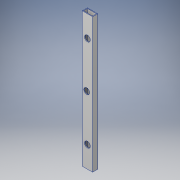
# Autodesk Inventor part: 26in 2x1
Saved by Autodesk Inventor 2018 (Build 220112000, 112)
## iProperties
Created: 2018-01-13
Part Number: 26in 2x1
Material: Aluminum 6061
Document SubType Name: Modeling
Designer: maste
Density: 2.7 g/cm^3
Appearance: Aluminum - Flat
Author: maste
Autodesk Inventor part; units mm, degrees
ref_plane "YZ Plane" through (0, 0, 0) normal (1, 0, 0) x (0, 1, 0)
ref_plane "XZ Plane" through (0, 0, 0) normal (0, 1, 0) x (-1, 0, 0)
ref_plane "XY Plane" through (0, 0, 0) normal (0, 0, 1) x (1, 0, 0)
sketch "Sketch1" plane through (0, 0, 0) normal (0, 1, 0) x (-1, 0, 0)
  line L0 (0, 0) -> (-50.8, 0)
  line L1 (-50.8, 0) -> (-50.8, -25.4)
  line L2 (-50.8, -25.4) -> (0, -25.4)
  line L3 (0, -25.4) -> (0, 0)
  line L4 (-3.175, -22.225) -> (-47.625, -22.225)
  line L5 (-47.625, -22.225) -> (-47.625, -3.175)
  line L6 (-47.625, -3.175) -> (-3.175, -3.175)
  line L7 (-3.175, -3.175) -> (-3.175, -22.225)
  dimension "d0" = 50.8
  dimension "d1" = 25.4
  dimension "d2" = 3.175
  dimension "d3" = 3.175
  dimension "d4" = 3.175
  dimension "d5" = 3.175
  constraints: 16 end point, 4 parallel, 2 horizontal, 2 perpendicular
  measures "d0" distance of L1.end L2.end
  measures "d1" distance of L0.end L1.end
  measures "d2" distance between parallel lines of L2 L4
  measures "d3" distance between parallel lines of L0 L6
  measures "d4" distance between parallel lines of L1 L5
  measures "d5" distance between parallel lines of L3 L7
extrude "Extrusion1" add sketch "Sketch1" along normal blind 660.4
sketch "Sketch2" plane through (0, 0, 0) normal (0, 0, 1) x (1, 0, 0)
  line L0 (3.175, 660.4) -> (47.625, 660.4) projected
  line L1 (25.4, 660.4) -> (25.4, 0)
  line L2 (25.4, 0) -> (25.4, 330.2)
  line L3 (25.4, 330.2) -> (22.225, 330.2)
  circle A0 centre (22.225, 330.2) radius 14.2875
  point P0 (0, 0)
  dimension "d11" = 3.175
  constraints: 6 end point, 2 coincident, 2 midpoint, 1 centre point, 1 horizontal, 1 perpendicular
  measures "d11" distance of L3.start L3.end
extrude "Extrusion2" cut sketch "Sketch2" against normal blind 25.4
sketch "Sketch3" plane through (0, 0, 0) normal (0, 0, 1) x (1, 0, 0)
  line L0 (0, 0) -> (50.8, 0) projected
  line L1 (25.4, 0) -> (25.4, 660.4)
  line L2 (0, 660.4) -> (50.8, 660.4) projected
  line L3 (25.4, 660.4) -> (25.4, 571.5)
  line L4 (25.4, 0) -> (25.4, 88.9)
  line L5 (25.4, 571.5) -> (25.4, 555.625)
  circle A0 centre (25.4, 555.625) radius 14.2875
  line L6 (25.4, 88.9) -> (25.4, 104.775)
  circle A1 centre (25.4, 104.775) radius 14.2875
  dimension "d12" = 88.9
  dimension "d13" = 88.9
  dimension "d17" = 15.875
  dimension "d18" = 15.875
  constraints: 10 end point, 4 coincident, 4 point on line, 2 centre point, 2 midpoint
  measures "d12" distance of L1.end L3.end
  measures "d13" distance of L1.start L4.end
  measures "d17" distance of L5.start L5.end
  measures "d18" distance of L6.start L6.end
extrude "Extrusion3" cut sketch "Sketch3" against normal blind 25.4
body "Solid1"
